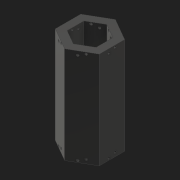
# Autodesk Inventor part: A01
Saved by Autodesk Inventor 2017 (Build 210142000, 142)
## iProperties
Created: 2019-09-19
Part Number: A01
Material: ABS Plastic
Document SubType Name: Modeling
Designer: Dell
Density: 1.06 g/cm^3
Appearance: Smooth - Black
Mass: 2688.13 g
Surface Area: 1514.93 cm^2
Volume: 2535.97 cm^3
Author: Dell
Autodesk Inventor part; units mm, degrees
ref_plane "YZ Plane" through (0, 0, 0) normal (1, 0, 0) x (0, 1, 0)
ref_plane "XZ Plane" through (0, 0, 0) normal (0, 1, 0) x (-1, 0, 0)
ref_plane "XY Plane" through (0, 0, 0) normal (0, 0, 1) x (1, 0, 0)
sketch "Sketch1" plane through (0, 0, 0) normal (0, 0, 1) x (1, 0, 0)
  line L0 (0, 57.735) -> (50, 28.8675)
  line L1 (50, 28.8675) -> (50, -28.8675)
  line L2 (50, -28.8675) -> (0, -57.735)
  line L3 (0, -57.735) -> (-50, -28.8675)
  line L4 (-50, -28.8675) -> (-50, 28.8675)
  line L5 (-50, 28.8675) -> (0, 57.735)
  line L6 (0, 38.1051) -> (33, 19.0526)
  line L7 (33, 19.0526) -> (33, -19.0526)
  line L8 (33, -19.0526) -> (0, -38.1051)
  line L9 (0, -38.1051) -> (-33, -19.0526)
  line L10 (-33, -19.0526) -> (-33, 19.0526)
  line L11 (-33, 19.0526) -> (0, 38.1051)
  point P0 (0, 0)
  point P1 (0, 0)
  dimension "d0" = 100
  dimension "d1" = 66
  constraints: 24 end point, 1 coincident, 1 vertical alignment, 18 other
  measures "d0" distance between parallel lines of L1 L4
  measures "d1" distance between parallel lines of L7 L10
extrude "Extrusion1" add sketch "Sketch1" along normal blind 220
sketch "Sketch2" plane through (50, -28.8675, 0) normal (1, 0, 0) x (0, 0, -1)
  line L0 (-211, 21.7964) -> (-216, 35.9386) construction
  line L1 (-220, 0) -> (-220, 57.735) projected
  circle A0 centre (-216, 35.9386) radius 2.5
  circle A1 centre (-211, 21.7964) radius 2.5
  line L2 (-4, 21.7964) -> (-9, 35.9386) construction
  circle A2 centre (-9, 35.9386) radius 2.5
  circle A3 centre (-4, 21.7964) radius 2.5
  line L3 (0, 57.735) -> (0, 0) projected
  point P0 (0, 28.8675)
  point P1 (-213.5, 28.8675)
  point P2 (-220, 28.8675)
  point P3 (-6.5, 28.8675)
  point P4 (0, 28.8675)
  dimension "d4" = 15
  dimension "d6" = 5
  dimension "d7" = 5
  dimension "d28" = 6.5
  dimension "d29" = 5
  dimension "d30" = 15
  dimension "d31" = 5
  dimension "d32" = 5
  dimension "d34" = 5
  dimension "d35" = 6.5
  constraints: 4 centre point, 4 coincident, 4 end point, 4 midpoint, 2 horizontal alignment
  measures "d4" distance of L0.start L0.end
  measures "d6" diameter of A0
  measures "d7" diameter of A1
  measures "d28" distance of point (-220, 28.868) point (-213.5, 28.868)
  measures "d29" horizontal distance of L0.start L0.end
  measures "d30" distance of L2.start L2.end
  measures "d31" diameter of A2
  measures "d32" diameter of A3
  measures "d34" horizontal distance of L2.start L2.end
  measures "d35" distance of point (0, 28.868) point (-6.5, 28.868)
extrude "Extrusion2" cut sketch "Sketch2" against normal blind 30
pattern_circular "Circular Pattern1" count 6 over 360 about axis through (0, 0, -10) along (0, 0, 1) of "Extrusion2"
body "Solid1"
